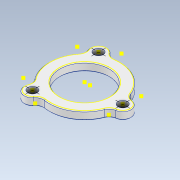
# Autodesk Inventor part: ServoBBLid
Saved by Autodesk Inventor 2020 (Build 240168000, 168)
## iProperties
Created: 2019-12-15
Part Number: ServoBBLid
Material: Aluminum 6061
Document SubType Name: Modeling
Designer: Kjell
Density: 2.7 g/cm^3
Appearance: Aluminum - Flat
Author: Kjell
Autodesk Inventor part; units mm, degrees
ref_plane "YZ Plane" through (0, 0, 0) normal (1, 0, 0) x (0, 1, 0)
ref_plane "XZ Plane" through (0, 0, 0) normal (0, 1, 0) x (-1, 0, 0)
ref_plane "XY Plane" through (0, 0, 0) normal (0, 0, 1) x (1, 0, 0)
ref_plane "Work Plane1" through (0, 0, 0) normal (0, 0, 1) x (1, 0, 0)
sketch "Sketch1" plane through (0, 0, 0) normal (0, 0, 1) x (1, 0, 0)
  circle A0 centre (-2, 0) radius 10.525
  circle A1 centre (-2, 0) radius 9
  arc A2 (-11.9786, 7.8561) -> (-11.9786, -7.8561) centre (-2, 0) ccw
  arc A3 (-11.5071, -11.1222) -> (-11.9786, -7.8561) centre (-14.5714, -9.8974) ccw
  arc A4 (-11.5071, -11.1222) -> (-6.8786, -13.7945) centre (-9, -12.1244) ccw
  arc A5 (-3.8143, -12.5697) -> (-6.8786, -13.7945) centre (-4.2857, -15.8359) ccw
  arc A6 (-3.8143, -12.5697) -> (9.7929, -4.7137) centre (-2, 0) ccw
  arc A7 (12.3857, -2.6723) -> (9.7929, -4.7137) centre (12.8571, -5.9385) ccw
  arc A8 (12.3857, -2.6723) -> (12.3857, 2.6723) centre (12, 0) ccw
  arc A9 (9.7929, 4.7137) -> (12.3857, 2.6723) centre (12.8571, 5.9385) ccw
  arc A10 (9.7929, 4.7137) -> (-3.8143, 12.5697) centre (-2, 0) ccw
  arc A11 (-6.8786, 13.7945) -> (-3.8143, 12.5697) centre (-4.2857, 15.8359) ccw
  arc A12 (-6.8786, 13.7945) -> (-11.5071, 11.1222) centre (-9, 12.1244) ccw
  arc A13 (-11.9786, 7.8561) -> (-11.5071, 11.1222) centre (-14.5714, 9.8974) ccw
  circle A14 centre (9, -14) radius 2.55
  circle A15 centre (-31, -14) radius 2.55
  arc A16 (-12.2143, 8.0417) -> (-11.7857, 11.0109) centre (-14.5714, 9.8974) ccw
  arc A17 (-6.6429, 13.9801) -> (-11.7857, 11.0109) centre (-9, 12.1244) ccw
  arc A18 (-6.6429, 13.9801) -> (-3.8571, 12.8667) centre (-4.2857, 15.8359) ccw
  arc A19 (10.0714, 4.825) -> (-3.8571, 12.8667) centre (-2, 0) ccw
  arc A20 (10.0714, 4.825) -> (12.4286, 2.9692) centre (12.8571, 5.9385) ccw
  arc A21 (12.4286, -2.9692) -> (12.4286, 2.9692) centre (12, 0) ccw
  arc A22 (12.4286, -2.9692) -> (10.0714, -4.825) centre (12.8571, -5.9385) ccw
  arc A23 (-3.8571, -12.8667) -> (10.0714, -4.825) centre (-2, 0) ccw
  arc A24 (-3.8571, -12.8667) -> (-6.6429, -13.9801) centre (-4.2857, -15.8359) ccw
  arc A25 (-11.7857, -11.0109) -> (-6.6429, -13.9801) centre (-9, -12.1244) ccw
  arc A26 (-11.7857, -11.0109) -> (-12.2143, -8.0417) centre (-14.5714, -9.8974) ccw
  arc A27 (-12.2143, 8.0417) -> (-12.2143, -8.0417) centre (-2, 0) ccw
  line L0 (-39.7, -19) -> (-39.7, 19)
  arc A28 (-39.7, -19) -> (-39, -19.7) centre (-39, -19) ccw
  line L1 (17, -19.7) -> (-39, -19.7)
  arc A29 (17, -19.7) -> (17.7, -19) centre (17, -19) ccw
  line L2 (17.7, 19) -> (17.7, -19)
  arc A30 (17.7, 19) -> (17, 19.7) centre (17, 19) ccw
  line L3 (-39, 19.7) -> (17, 19.7)
  arc A31 (-39, 19.7) -> (-39.7, 19) centre (-39, 19) ccw
  circle A32 centre (-31, 14) radius 2.55
  circle A33 centre (9, 14) radius 2.55
  point P0 (0, 0)
  dimension "d0" = 18
  constraints: 56 point on circle, 34 centre point, 8 end point, 1 coincident
  measures "d0" diameter of A1
extrude "Extrusion2" add sketch "Sketch1" along normal blind 3 contours A0 | A13 A12 A11 A10 A9 A8 A7 A6 A5 A4 A3 A2 | A16 A17 A18 A19 A20 A21 A22 A23 A24 A25 A26 A27
chamfer "Chamfer2" distance 0.3 angle 45 26 edges at (-15, 0, 3) (-11.6022, -9.4689, 3) (-10.5, -14.7224, 3) (-5.3992, -13.0502, 3) (4.5, -11.2583, 3) (11.0014, -3.5813, 3) (15, 0, 3) (11.0014, 3.5813, 3) (4.5, 11.2583, 3) (-5.3992, 13.0502, 3) (-10.5, 14.7224, 3) (-11.6022, 9.4689, 3) (-11, 0, 3) (-11, 0, 0) (4.5, -11.2583, 0) (11.0014, -3.5813, 0) (15, 0, 0) (11.0014, 3.5813, 0) (4.5, 11.2583, 0) (-5.3992, 13.0502, 0) (-10.5, 14.7224, 0) (-11.6022, 9.4689, 0) (-15, 0, 0) (-11.6022, -9.4689, 0) (-10.5, -14.7224, 0) (-5.3992, -13.0502, 0)
sketch "Sketch4" plane through (0, 0, 3) normal (0, 0, 1) x (1, 0, 0)
  arc A0 (-11.9786, 7.8561) -> (-11.9786, -7.8561) centre (-2, 0) ccw projected
  arc A1 (-11.5071, -11.1222) -> (-11.9786, -7.8561) centre (-14.5714, -9.8974) ccw projected
  arc A2 (-11.5071, -11.1222) -> (-6.8786, -13.7945) centre (-9, -12.1244) ccw projected
  arc A3 (-3.8143, -12.5697) -> (-6.8786, -13.7945) centre (-4.2857, -15.8359) ccw projected
  arc A4 (-3.8143, -12.5697) -> (9.7929, -4.7137) centre (-2, 0) ccw projected
  arc A5 (12.3857, -2.6723) -> (9.7929, -4.7137) centre (12.8571, -5.9385) ccw projected
  arc A6 (12.3857, -2.6723) -> (12.3857, 2.6723) centre (12, 0) ccw projected
  arc A7 (9.7929, 4.7137) -> (12.3857, 2.6723) centre (12.8571, 5.9385) ccw projected
  arc A8 (9.7929, 4.7137) -> (-3.8143, 12.5697) centre (-2, 0) ccw projected
  arc A9 (-6.8786, 13.7945) -> (-3.8143, 12.5697) centre (-4.2857, 15.8359) ccw projected
  arc A10 (-6.8786, 13.7945) -> (-11.5071, 11.1222) centre (-9, 12.1244) ccw projected
  arc A11 (-11.9786, 7.8561) -> (-11.5071, 11.1222) centre (-14.5714, 9.8974) ccw projected
  circle A12 centre (-2, 0) radius 9.3 projected
  point P0 (0, 0)
  constraints: 3 coincident
sketch "Sketch5" plane through (0, 0, 3) normal (0, 0, 1) x (1, 0, 0)
  point P0 (12, 0)
  point P1 (-9, -12.1244)
  point P2 (-9, 12.1244)
hole "Hole1" at (12, 0, 3) at (-9, -12.1244, 3) at (-9, 12.1244, 3) direction (0, 0, -1) diameter 3.4 depth 3
body "Solid2"
